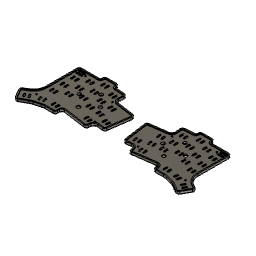
MUSUBI_V2_CASE_SOLID (Autodesk Fusion 360 design; units mm, degrees)
Autodesk Fusion 360 part; units mm, degrees
sketch "WIP_case_bottom" plane through (0, 0, 0) normal (0, 0, 1) x (1, 0, 0)
  arc A0 (118.3392, 82.5249) -> (115.7392, 82.5249) centre (117.0392, 82.5249) ccw
  arc A1 (44.5211, 69.8152) -> (47.0958, 70.177) centre (45.8084, 69.9961) cw
  line L0 (97.2392, 72.1249) -> (97.2392, 67.21)
  line L1 (85.5392, 93.21) -> (85.5392, 98.1249)
  line L2 (134.3532, 17.2954) -> (131.8958, 13.039)
  arc A2 (41.0427, 45.7043) -> (43.6174, 46.0661) centre (42.3301, 45.8852) ccw
  arc A3 (59.8359, 47.9392) -> (62.4296, 48.1205) centre (61.1327, 48.0298) ccw
  line L3 (92.9859, 25.8609) -> (92.9859, 20.9461)
  line L4 (99.7859, 20.9461) -> (99.7859, 25.8609)
  arc A4 (122.5392, 45.5377) -> (125.1392, 45.5377) centre (123.8392, 45.5377) cw
  arc A5 (22.857, 38.5814) -> (25.4317, 38.9432) centre (24.1444, 38.7623) ccw
  arc A6 (88.1392, 56.2105) -> (85.5392, 56.2105) centre (86.8392, 56.2105) cw
  arc A7 (122.5392, 82.5249) -> (125.1392, 82.5249) centre (123.8392, 82.5249) cw
  line L5 (88.1392, 79.6249) -> (88.1392, 74.71)
  line L6 (118.3392, 77.61) -> (118.3392, 82.5249)
  arc A8 (118.3392, 64.0249) -> (115.7392, 64.0249) centre (117.0392, 64.0249) ccw
  line L7 (65.3312, 66.834) -> (64.9884, 71.7369)
  line L8 (104.0392, 48.9605) -> (104.0392, 53.8754)
  arc A9 (125.1392, 59.11) -> (122.5392, 59.11) centre (123.8392, 59.11) cw
  line L9 (106.6392, 53.8754) -> (106.6392, 48.9605)
  line L10 (78.7392, 79.6249) -> (78.7392, 74.71)
  arc A10 (57.2561, 84.8317) -> (59.8498, 85.013) centre (58.5529, 84.9223) ccw
  line L11 (99.8392, 85.71) -> (99.8392, 90.6249)
  arc A11 (95.5859, 25.8609) -> (92.9859, 25.8609) centre (94.2859, 25.8609) ccw
  arc A12 (104.0392, 53.8754) -> (106.6392, 53.8754) centre (105.3392, 53.8754) cw
  arc A13 (140.0364, 8.339) -> (137.7847, 9.639) centre (138.9106, 8.989) cw
  arc A14 (45.5088, 32.6083) -> (42.9341, 32.2464) centre (44.2215, 32.4273) ccw
  line L12 (81.3392, 74.71) -> (81.3392, 79.6249)
  line L13 (52.2427, 33.5546) -> (52.9267, 28.6876)
  arc A15 (102.3859, 20.9461) -> (99.7859, 20.9461) centre (101.0859, 20.9461) cw
  line L14 (61.1415, 66.541) -> (60.7986, 71.4439)
  arc A16 (120.8016, 22.5413) -> (123.313, 21.8684) centre (122.0573, 22.2048) cw
  line L15 (62.4296, 48.1205) -> (62.0867, 53.0234)
  arc A17 (67.9249, 67.0154) -> (65.3312, 66.834) centre (66.6281, 66.9247) cw
  line L16 (78.7392, 98.1249) -> (78.7392, 93.21)
  arc A18 (59.5069, 89.9159) -> (56.9132, 89.7345) centre (58.2101, 89.8252) ccw
  line L17 (118.3392, 59.11) -> (118.3392, 64.0249)
  arc A19 (99.7859, 25.8609) -> (102.3859, 25.8609) centre (101.0859, 25.8609) cw
  arc A20 (115.7392, 40.6228) -> (118.3392, 40.6228) centre (117.0392, 40.6228) ccw
  line L18 (125.1392, 45.5377) -> (125.1392, 40.6228)
  line L19 (104.0392, 67.21) -> (104.0392, 72.1249)
  line L20 (59.8498, 85.013) -> (59.5069, 89.9159)
  arc A21 (140.2422, 13.8954) -> (142.4938, 12.5954) centre (141.368, 13.2454) cw
  line L21 (67.582, 71.9183) -> (67.9249, 67.0154)
  line L22 (43.6174, 46.0661) -> (42.9334, 50.9332)
  line L23 (41.0459, 64.3636) -> (40.3619, 69.2307)
  line L24 (106.6392, 90.6249) -> (106.6392, 85.71)
  line L25 (88.1392, 98.1249) -> (88.1392, 93.21)
  line L26 (99.8392, 48.9605) -> (99.8392, 53.8754)
  arc A22 (64.9884, 71.7369) -> (67.582, 71.9183) centre (66.2852, 71.8276) cw
  line L27 (106.6392, 72.1249) -> (106.6392, 67.21)
  line L28 (125.1392, 82.5249) -> (125.1392, 77.61)
  arc A23 (78.7392, 56.2105) -> (81.3392, 56.2105) centre (80.0392, 56.2105) ccw
  line L29 (95.5859, 20.9461) -> (95.5859, 25.8609)
  line L30 (102.3859, 25.8609) -> (102.3859, 20.9461)
  line L31 (99.8392, 67.21) -> (99.8392, 72.1249)
  line L32 (64.0395, 85.306) -> (63.6967, 90.2089)
  line L33 (46.1928, 27.7412) -> (45.5088, 32.6083)
  arc A24 (63.6967, 90.2089) -> (66.2903, 90.3903) centre (64.9935, 90.2996) cw
  line L34 (85.5392, 56.2105) -> (85.5392, 61.1254)
  arc A25 (66.2765, 53.3164) -> (68.8701, 53.4978) centre (67.5733, 53.4071) cw
  line L35 (115.7392, 45.5377) -> (115.7392, 40.6228)
  line L36 (137.7847, 9.639) -> (140.2422, 13.8954)
  arc A26 (58.5478, 66.3597) -> (61.1415, 66.541) centre (59.8446, 66.4503) ccw
  line L37 (22.173, 43.4484) -> (22.857, 38.5814)
  arc A27 (112.9613, 19.5538) -> (115.4727, 18.8809) centre (114.217, 19.2174) ccw
  arc A28 (52.9267, 28.6876) -> (50.352, 28.3257) centre (51.6393, 28.5067) cw
  arc A29 (88.1392, 74.71) -> (85.5392, 74.71) centre (86.8392, 74.71) cw
  line L38 (97.2392, 90.6249) -> (97.2392, 85.71)
  line L39 (115.7392, 64.0249) -> (115.7392, 59.11)
  arc A30 (62.0867, 53.0234) -> (59.493, 52.842) centre (60.7899, 52.9327) ccw
  arc A31 (104.0392, 90.6249) -> (106.6392, 90.6249) centre (105.3392, 90.6249) cw
  line L40 (42.9341, 32.2464) -> (43.6181, 27.3794)
  arc A32 (47.0926, 51.5177) -> (49.6673, 51.8795) centre (48.3799, 51.6986) cw
  line L41 (85.5392, 74.71) -> (85.5392, 79.6249)
  arc A33 (69.213, 48.5949) -> (66.6193, 48.4135) centre (67.9162, 48.5042) cw
  line L42 (104.0392, 85.71) -> (104.0392, 90.6249)
  line L43 (25.4317, 38.9432) -> (24.7477, 43.8102)
  arc A34 (78.7392, 93.21) -> (81.3392, 93.21) centre (80.0392, 93.21) ccw
  arc A35 (118.3392, 45.5377) -> (115.7392, 45.5377) centre (117.0392, 45.5377) ccw
  arc A36 (49.668, 33.1928) -> (52.2427, 33.5546) centre (50.9553, 33.3737) cw
  arc A37 (88.1392, 93.21) -> (85.5392, 93.21) centre (86.8392, 93.21) cw
  line L44 (59.493, 52.842) -> (59.8359, 47.9392)
  line L45 (122.5392, 77.61) -> (122.5392, 82.5249)
  arc A38 (85.5392, 61.1254) -> (88.1392, 61.1254) centre (86.8392, 61.1254) cw
  line L46 (97.2392, 53.8754) -> (97.2392, 48.9605)
  line L47 (66.2903, 90.3903) -> (66.6332, 85.4874)
  arc A39 (97.2392, 48.9605) -> (99.8392, 48.9605) centre (98.5392, 48.9605) ccw
  arc A40 (47.7798, 65.31) -> (45.2051, 64.9481) centre (46.4924, 65.1291) cw
  line L48 (115.7392, 82.5249) -> (115.7392, 77.61)
  line L49 (66.6193, 48.4135) -> (66.2765, 53.3164)
  arc A41 (106.6392, 67.21) -> (104.0392, 67.21) centre (105.3392, 67.21) cw
  arc A42 (40.3619, 69.2307) -> (37.7872, 68.8688) centre (39.0746, 69.0497) ccw
  line L50 (115.4727, 18.8809) -> (116.7447, 23.6283)
  arc A43 (106.6392, 48.9605) -> (104.0392, 48.9605) centre (105.3392, 48.9605) cw
  arc A44 (125.1392, 77.61) -> (122.5392, 77.61) centre (123.8392, 77.61) cw
  line L51 (122.5392, 59.11) -> (122.5392, 64.0249)
  line L52 (119.5296, 17.7939) -> (120.8016, 22.5413)
  arc A45 (81.3392, 79.6249) -> (78.7392, 79.6249) centre (80.0392, 79.6249) ccw
  arc A46 (85.5392, 98.1249) -> (88.1392, 98.1249) centre (86.8392, 98.1249) cw
  arc A47 (99.8392, 90.6249) -> (97.2392, 90.6249) centre (98.5392, 90.6249) ccw
  arc A48 (115.7392, 77.61) -> (118.3392, 77.61) centre (117.0392, 77.61) ccw
  line L53 (142.4938, 12.5954) -> (140.0364, 8.339)
  line L54 (56.9132, 89.7345) -> (57.2561, 84.8317)
  arc A49 (122.5392, 64.0249) -> (125.1392, 64.0249) centre (123.8392, 64.0249) cw
  arc A50 (115.7392, 59.11) -> (118.3392, 59.11) centre (117.0392, 59.11) ccw
  line L55 (114.2333, 24.3012) -> (112.9613, 19.5538)
  arc A51 (81.3392, 98.1249) -> (78.7392, 98.1249) centre (80.0392, 98.1249) ccw
  line L56 (68.8701, 53.4978) -> (69.213, 48.5949)
  line L57 (81.3392, 56.2105) -> (81.3392, 61.1254)
  arc A52 (32.1656, 39.8896) -> (29.5909, 39.5277) centre (30.8782, 39.7086) cw
  arc A53 (24.7477, 43.8102) -> (22.173, 43.4484) centre (23.4604, 43.6293) ccw
  arc A54 (97.2392, 85.71) -> (99.8392, 85.71) centre (98.5392, 85.71) ccw
  arc A55 (116.7447, 23.6283) -> (114.2333, 24.3012) centre (115.489, 23.9648) ccw
  line L58 (47.7766, 46.6506) -> (47.0926, 51.5177)
  arc A56 (66.6332, 85.4874) -> (64.0395, 85.306) centre (65.3364, 85.3967) cw
  arc A57 (104.0392, 72.1249) -> (106.6392, 72.1249) centre (105.3392, 72.1249) cw
  line L59 (45.2051, 64.9481) -> (44.5211, 69.8152)
  arc A58 (99.8392, 72.1249) -> (97.2392, 72.1249) centre (98.5392, 72.1249) ccw
  arc A59 (38.4712, 64.0018) -> (41.0459, 64.3636) centre (39.7586, 64.1827) ccw
  arc A60 (42.9334, 50.9332) -> (40.3587, 50.5713) centre (41.6461, 50.7522) ccw
  line L60 (125.1392, 64.0249) -> (125.1392, 59.11)
  line L61 (40.3587, 50.5713) -> (41.0427, 45.7043)
  arc A61 (92.9859, 20.9461) -> (95.5859, 20.9461) centre (94.2859, 20.9461) ccw
  line L62 (31.4816, 44.7566) -> (32.1656, 39.8896)
  line L63 (118.3392, 40.6228) -> (118.3392, 45.5377)
  arc A62 (122.041, 17.121) -> (119.5296, 17.7939) centre (120.7853, 17.4574) cw
  arc A63 (97.2392, 67.21) -> (99.8392, 67.21) centre (98.5392, 67.21) ccw
  arc A64 (43.6181, 27.3794) -> (46.1928, 27.7412) centre (44.9055, 27.5603) ccw
  line L64 (47.0958, 70.177) -> (47.7798, 65.31)
  arc A65 (60.7986, 71.4439) -> (58.2049, 71.2625) centre (59.5018, 71.3532) ccw
  line L65 (88.1392, 61.1254) -> (88.1392, 56.2105)
  arc A66 (106.6392, 85.71) -> (104.0392, 85.71) centre (105.3392, 85.71) cw
  line L66 (37.7872, 68.8688) -> (38.4712, 64.0018)
  arc A67 (78.7392, 74.71) -> (81.3392, 74.71) centre (80.0392, 74.71) ccw
  line L67 (58.2049, 71.2625) -> (58.5478, 66.3597)
  line L68 (122.5392, 40.6228) -> (122.5392, 45.5377)
  line L69 (50.352, 28.3257) -> (49.668, 33.1928)
  arc A68 (81.3392, 61.1254) -> (78.7392, 61.1254) centre (80.0392, 61.1254) ccw
  line L70 (78.7392, 61.1254) -> (78.7392, 56.2105)
  arc A69 (50.3513, 47.0125) -> (47.7766, 46.6506) centre (49.0639, 46.8316) cw
  arc A70 (131.8958, 13.039) -> (134.1474, 11.739) centre (133.0216, 12.389) ccw
  line L71 (29.5909, 39.5277) -> (28.9069, 44.3948)
  arc A71 (28.9069, 44.3948) -> (31.4816, 44.7566) centre (30.1942, 44.5757) cw
  arc A72 (125.1392, 40.6228) -> (122.5392, 40.6228) centre (123.8392, 40.6228) cw
  arc A73 (99.8392, 53.8754) -> (97.2392, 53.8754) centre (98.5392, 53.8754) ccw
  line L72 (134.1474, 11.739) -> (136.6049, 15.9954)
  line L73 (81.3392, 93.21) -> (81.3392, 98.1249)
  arc A74 (136.6049, 15.9954) -> (134.3532, 17.2954) centre (135.479, 16.6454) ccw
  line L74 (49.6673, 51.8795) -> (50.3513, 47.0125)
  arc A75 (85.5392, 79.6249) -> (88.1392, 79.6249) centre (86.8392, 79.6249) cw
  line L75 (123.313, 21.8684) -> (122.041, 17.121)
  arc A76 (149.9758, 14.4546) -> (149.2438, 17.1867) centre (148.2438, 15.4546) ccw
  arc A77 (38.4354, 24.3772) -> (29.4001, 31.1861) centre (30.5133, 23.2639) ccw
  line L76 (35.0406, 32.149) -> (36.3397, 29.899)
  circle A78 centre (92.8808, 60.1463) radius 3.2
  line L77 (97.6892, 97.976) -> (128.6892, 97.976)
  line L78 (131.4373, 20.399) -> (132.7363, 22.649)
  line L79 (50.8392, 75.1493) -> (53.4373, 75.1493)
  circle A79 centre (114.7682, 92.976) radius 1.3
  line L80 (36.3397, 34.399) -> (35.0406, 32.149)
  line L81 (128.8392, 24.899) -> (127.5401, 22.649)
  line L82 (53.4373, 79.6493) -> (50.8392, 79.6493)
  line L83 (141.7258, 0.1652) -> (149.9758, 14.4546)
  line L84 (41.2571, 18.6704) -> (80.6009, 24.1996)
  arc A80 (130.6892, 95.976) -> (128.6892, 97.976) centre (128.6892, 95.976) ccw
  line L85 (40.2368, 32.149) -> (38.9378, 34.399)
  arc A81 (93.6892, 101.976) -> (97.6892, 97.976) centre (97.6892, 101.976) ccw
  arc A82 (87.4359, 18.258) -> (80.6009, 24.1996) centre (81.4359, 18.258) ccw
  line L86 (38.9982, 20.3726) -> (38.4354, 24.3772)
  line L87 (36.3397, 29.899) -> (38.9378, 29.899)
  line L88 (127.7922, 89.3705) -> (119.0802, 89.3705)
  arc A83 (119.0802, 96.576) -> (119.0802, 93.976) centre (119.0802, 95.276) ccw
  line L89 (121.0068, 8.8736) -> (109.7331, 11.8943)
  arc A84 (130.6892, 41.7555) -> (142.6892, 20.9709) centre (154.6892, 41.7555) ccw
  arc A85 (127.7922, 93.976) -> (127.7922, 96.576) centre (127.7922, 95.276) ccw
  line L90 (69.4682, 97.9815) -> (52.8591, 96.8201)
  line L91 (49.5401, 77.3993) -> (50.8392, 75.1493)
  line L92 (73.1892, 101.9718) -> (73.1892, 103.476)
  line L93 (138.9938, -0.5669) -> (126.7953, 6.4759)
  line L94 (113.4692, 95.226) -> (112.1701, 92.976)
  line L95 (149.2438, 17.1867) -> (142.6892, 20.9709)
  circle A86 centre (73.1925, 78.5273) radius 3.2
  arc A87 (109.7331, 11.8943) -> (103.5216, 12.712) centre (103.5216, -11.288) ccw
  arc A88 (75.1892, 105.476) -> (73.1892, 103.476) centre (75.1892, 103.476) ccw
  line L96 (127.7922, 96.576) -> (119.0802, 96.576)
  line L97 (132.7363, 22.649) -> (131.4373, 24.899)
  circle A89 centre (74.5198, 40.4393) radius 3.2
  arc A90 (87.4359, 14.712) -> (89.4359, 12.712) centre (89.4359, 14.712) ccw
  line L98 (29.4001, 31.1861) -> (20.4874, 29.9337)
  line L99 (38.9378, 29.899) -> (40.2368, 32.149)
  line L100 (112.1701, 92.976) -> (113.4692, 90.726)
  arc A91 (127.7922, 91.9705) -> (127.7922, 89.3705) centre (127.7922, 90.6705) cw
  circle A92 centre (52.1382, 77.3993) radius 1.3
  line L101 (54.7363, 77.3993) -> (53.4373, 79.6493)
  line L102 (127.5401, 22.649) -> (128.8392, 20.399)
  line L103 (44.761, 77.2722) -> (14.4336, 73.0101)
  line L104 (75.1892, 105.476) -> (91.6892, 105.476)
  arc A93 (93.6892, 103.476) -> (91.6892, 105.476) centre (91.6892, 103.476) ccw
  line L105 (119.0802, 91.9705) -> (127.7922, 91.9705)
  line L106 (38.9378, 34.399) -> (36.3397, 34.399)
  circle A94 centre (130.1382, 22.649) radius 1.3
  line L107 (117.3663, 92.976) -> (116.0673, 95.226)
  line L108 (93.6892, 103.476) -> (93.6892, 101.976)
  line L109 (130.6892, 41.7555) -> (130.6892, 95.976)
  circle A95 centre (54.8122, 58.8197) radius 3.2
  line L110 (116.0673, 95.226) -> (113.4692, 95.226)
  line L111 (53.4373, 75.1493) -> (54.7363, 77.3993)
  arc A96 (69.4682, 97.9815) -> (73.1892, 101.9718) centre (69.1892, 101.9718) ccw
  arc A97 (44.761, 77.2722) -> (51.6282, 85.7524) centre (43.6476, 85.1944) ccw
  arc A98 (52.8591, 96.8201) -> (51.0035, 94.6855) centre (52.9986, 94.825) ccw
  circle A99 centre (73.8502, 59.4845) radius 20.55
  line L112 (116.0673, 90.726) -> (117.3663, 92.976)
  line L113 (50.8392, 79.6493) -> (49.5401, 77.3993)
  line L114 (87.4359, 14.712) -> (87.4359, 18.258)
  line L115 (12.9472, 69.2162) -> (12.7314, 70.7512)
  line L116 (113.4692, 90.726) -> (116.0673, 90.726)
  arc A100 (138.9938, -0.5669) -> (141.7258, 0.1652) centre (139.9938, 1.1652) ccw
  line L117 (119.0802, 93.976) -> (127.7922, 93.976)
  arc A101 (14.4336, 73.0101) -> (12.7314, 70.7512) centre (14.712, 71.0296) ccw
  arc A102 (119.0802, 89.3705) -> (119.0802, 91.9705) centre (119.0802, 90.6705) cw
  arc A103 (38.9982, 20.3726) -> (41.2571, 18.6704) centre (40.9788, 20.6509) ccw
  arc A104 (126.7953, 6.4759) -> (121.0068, 8.8736) centre (114.7953, -14.3087) ccw
  line L118 (131.4373, 24.899) -> (128.8392, 24.899)
  line L119 (51.6282, 85.7524) -> (51.0035, 94.6855)
  circle A105 centre (37.6387, 32.149) radius 1.3
  arc A106 (18.2286, 31.6359) -> (20.4874, 29.9337) centre (20.2091, 31.9142) ccw
  line L120 (103.5216, 12.712) -> (89.4359, 12.712)
  line L121 (128.8392, 20.399) -> (131.4373, 20.399)
  line L122 (95.6892, 103.476) -> (95.6892, 101.976)
  line L123 (12.9472, 69.2162) -> (18.2286, 31.6359)
  line L124 (29.6784, 29.2056) -> (20.7658, 27.9532)
  arc A107 (16.2481, 31.3576) -> (20.7658, 27.9532) centre (20.2091, 31.9142) ccw
  line L125 (10.9666, 68.9379) -> (16.2481, 31.3576)
  line L126 (10.9666, 68.9379) -> (10.7509, 70.4729)
  arc A108 (14.1553, 74.9906) -> (10.7509, 70.4729) centre (14.712, 71.0296) ccw
  line L127 (44.4827, 79.2528) -> (14.1553, 74.9906)
  arc A109 (44.4827, 79.2528) -> (49.633, 85.6129) centre (43.6476, 85.1944) ccw
  line L128 (49.633, 85.6129) -> (49.0084, 94.5459)
  arc A110 (52.7196, 98.8152) -> (49.0084, 94.5459) centre (52.9986, 94.825) ccw
  line L129 (69.3287, 99.9767) -> (52.7196, 98.8152)
  arc A111 (69.3287, 99.9767) -> (71.1892, 101.9718) centre (69.1892, 101.9718) ccw
  line L130 (71.1892, 101.9718) -> (71.1892, 103.476)
  arc A112 (75.1892, 107.476) -> (71.1892, 103.476) centre (75.1892, 103.476) ccw
  line L131 (75.1892, 107.476) -> (91.6892, 107.476)
  arc A113 (95.6892, 103.476) -> (91.6892, 107.476) centre (91.6892, 103.476) ccw
  line L132 (95.6892, 103.476) -> (95.6892, 101.976)
  arc A114 (95.6892, 101.976) -> (97.6892, 99.976) centre (97.6892, 101.976) ccw
  line L133 (97.6892, 99.976) -> (128.6892, 99.976)
  arc A115 (132.6892, 95.976) -> (128.6892, 99.976) centre (128.6892, 95.976) ccw
  line L134 (132.6892, 41.7555) -> (132.6892, 95.976)
  arc A116 (132.6892, 41.7555) -> (143.6892, 22.703) centre (154.6892, 41.7555) ccw
  line L135 (150.2438, 18.9187) -> (143.6892, 22.703)
  arc A117 (151.7079, 13.4546) -> (150.2438, 18.9187) centre (148.2438, 15.4546) ccw
  line L136 (143.4579, -0.8348) -> (151.7079, 13.4546)
  arc A118 (137.9938, -2.2989) -> (143.4579, -0.8348) centre (139.9938, 1.1652) ccw
  line L137 (137.9938, -2.2989) -> (125.7953, 4.7439)
  arc A119 (125.7953, 4.7439) -> (120.4892, 6.9417) centre (114.7953, -14.3087) ccw
  line L138 (120.4892, 6.9417) -> (109.2155, 9.9624)
  arc A120 (109.2155, 9.9624) -> (103.5216, 10.712) centre (103.5216, -11.288) ccw
  line L139 (103.5216, 10.712) -> (89.4359, 10.712)
  arc A121 (85.4359, 14.712) -> (89.4359, 10.712) centre (89.4359, 14.712) ccw
  line L140 (85.4359, 14.712) -> (85.4359, 18.258)
  arc A122 (85.4359, 18.258) -> (80.8792, 22.2191) centre (81.4359, 18.258) ccw
  line L141 (41.5354, 16.6898) -> (80.8792, 22.2191)
  arc A123 (37.0177, 20.0942) -> (41.5354, 16.6898) centre (40.9788, 20.6509) ccw
  line L142 (37.0177, 20.0942) -> (36.4549, 24.0989)
  arc A124 (36.4549, 24.0989) -> (29.6784, 29.2056) centre (30.5133, 23.2639) ccw
  dimension "d28" = 2
  constraint tangent A106 L123
extrude "Extrude1" add sketch "WIP_case_bottom" along normal blind 4.6 contours L122 L124 A107 L125 L126 A108 L127 A109 L128 A110 L129 A111 L130 A112 L131 A113 L132 A114 L133 A115 L134 A116 L135 A117 L136 A118 L137 A119 L138 A120 L139 A121 L140 A122 L141 A123 L142 A124 makes body 1
extrude "Extrude2" add sketch "WIP_case_bottom" along normal blind 3 contours L10 L12 A29 L41 A67 A78 A86 A89 A95 A99 | A76 A77 L77 L83 L84 A80 A81 A82 L86 L89 A84 L90 L92 L93 L95 A87 A88 A90 L98 L103 L104 A93 L108 L109 A96 A97 A98 L114 L115 A100 A101 A103 A104 L119 A106 L120 L123 bodies 1
extrude "Extrude3" add sketch "WIP_case_bottom" along normal blind 1.5 contours A0 L6 L48 A48 | A1 A40 L59 L64 | L0 L31 A58 A63 | L1 L25 A37 A46 | L2 A70 L72 A74 | A2 L22 A60 L61 | A3 L15 A30 L44 | L3 A11 L29 A61 | L4 A15 A19 L30 | A4 L18 L68 A72 | A5 L37 L43 A53 | A6 L34 A38 L65 | A7 L28 L45 A44 | L5 A29 L41 A75 A99 | A29 L41 A99 | L10 L12 A45 A99 | L10 L12 A67 A99 | A8 L17 L39 A50 | L7 A17 L21 A22 | L8 L9 A12 A43 | A9 L51 A49 L60 | A10 A18 L20 L54 | L11 L38 A47 A54 | A13 A21 L36 L53 | A14 L33 L40 A64 | L13 A28 A36 L69 | L14 A26 A65 L67 | A16 L52 A62 L75 | L16 A34 A51 L73 | A20 L35 A35 L63 | L19 L27 A41 A57 | L23 A42 A59 L66 | L24 A31 L42 A66 | L26 L46 A39 A73 | A23 L57 A68 L70 | L32 A24 L47 A56 | A25 A33 L49 L56 | A27 L50 L55 A55 | A32 L58 A69 L74 | A52 L62 L71 A71 bodies 1
extrude "Extrude4" cut sketch "WIP_case_bottom" along normal blind 1 contours A3 L15 A30 L44 | A6 L34 A38 L65 | L10 L12 A29 L41 A67 A78 A86 A89 A95 A99 | A29 L41 A99 | L10 L12 A67 A99 | L7 A17 L21 A22 | L14 A26 A65 L67 | A23 L57 A68 L70 | A25 A33 L49 L56 bodies 1
extrude "Extrude5" add sketch "WIP_case_bottom" along normal blind 1.5 contours L88 A91 L105 A102 | A83 A85 L96 L117 bodies 1
extrude "Extrude6" add sketch "WIP_case_bottom" along normal blind 3 contours L76 L80 L85 L87 L99 L106 | L78 L81 L97 L102 L118 L121 | L79 L82 L91 L101 L111 L113 | A79 | L94 L100 L107 L110 L112 L116 | A92 | A94 | A105 bodies 1
extrude "Extrude7" cut sketch "WIP_case_bottom" along normal blind 3 contours A79 | A92 | A94 | A105 bodies 1
extrude "Extrude8" cut sketch "WIP_case_bottom" along normal blind 1.6 contours L76 L80 L85 L87 L99 L106 | L78 L81 L97 L102 L118 L121 | L79 L82 L91 L101 L111 L113 | L94 L100 L107 L110 L112 L116 bodies 1
chamfer "Chamfer1" distance 0.75 angle 45 36 edges at (49.9798, 97.4492, 0) (49.3207, 90.0794, 0) (48.3105, 81.4184, 0) (29.319, 77.1217, 0) (11.5174, 73.4368, 0) (13.4995, 50.9152, 0) (17.8018, 28.7197, 0) (25.2221, 28.5794, 0) (34.1242, 28.0557, 0) (36.7363, 22.0966, 0) (38.5715, 17.4564, 0) (61.2073, 19.4545, 0) (84.0601, 21.2769, 0) (85.4359, 16.485, 0) (86.6075, 11.8836, 0) (96.4788, 10.712, 0) (106.3931, 10.5238, 0) (114.8524, 8.4521, 0) (123.2143, 6.0167, 0) (131.8946, 1.2225, 0) (141.0291, -2.6985, 0) (147.5829, 6.3099, 0) (152.1075, 16.4899, 0) (146.9665, 20.8108, 0) (135.6367, 30.7556, 0) (132.6892, 68.8658, 0) (131.5176, 98.8044, 0) (113.1892, 99.976, 0) (96.275, 100.5618, 0) (95.6892, 102.726, 0) (94.5176, 106.3044, 0) (83.4392, 107.476, 0) (72.3608, 106.3044, 0) (71.1892, 102.7239, 0) (70.6519, 100.6078, 0) (61.0242, 99.396, 0) on bodies 1
mirror "Mirror1" about plane through (0, 0, 0) normal (1, 0, 0) of bodies 1 makes body 2
extrude "Extrude9" add 40 faces at (-87.2726, 57.8488, 1.5) (-79.6059, 57.8488, 1.5) (-86.4059, 76.3483, 1.5) (-79.6059, 77.9866, 1.5) (-80.4726, 94.8483, 1.5) (-86.4059, 96.4866, 1.5) (-98.1059, 87.3483, 1.5) (-105.7726, 87.3483, 1.5) (-104.9059, 70.4866, 1.5) (-98.1059, 70.4866, 1.5) (-117.4726, 79.2483, 1.5) (-123.4059, 79.2483, 1.5) (-124.2726, 60.7483, 1.5) (-116.6059, 60.7483, 1.5) (-121.9842, 91.1038, 1.5) (-121.9842, 95.7093, 1.5) (-98.1059, 50.5988, 1.5) (-105.7726, 52.2371, 1.5) (-117.4726, 42.2611, 1.5) (-124.2726, 42.2611, 1.5) (-140.105, 10.1912, 1.5) (-134.2846, 15.4433, 1.5) (-121.6279, 18.9277, 1.5) (-115.0596, 20.6877, 1.5) (-101.5192, 22.5843, 1.5) (-94.7192, 22.5843, 1.5) (-65.5401, 88.6955, 1.5) (-58.0064, 86.5264, 1.5) (-65.9672, 70.1631, 1.5) (-59.2981, 68.0544, 1.5) (-67.3696, 50.1083, 1.5) (-61.4507, 49.6944, 1.5) (-51.8404, 30.1893, 1.5) (-44.0204, 30.7447, 1.5) (-49.265, 48.5142, 1.5) (-41.445, 49.0696, 1.5) (-46.6935, 66.8117, 1.5) (-39.9597, 65.8653, 1.5) (-30.8513, 43.0136, 1.5) (-24.3455, 40.4449, 1.5) along direction (0, 0, 1) blind 0.5 on bodies 2 bodies 2
delete_body "RemoveBody1" bodies 2
extrude "Extrude10" add 40 faces at (24.3455, 40.4449, 1.5) (30.8513, 43.0136, 1.5) (44.0204, 30.7447, 1.5) (51.8404, 30.1893, 1.5) (41.445, 49.0696, 1.5) (49.265, 48.5142, 1.5) (39.9597, 65.8653, 1.5) (46.6935, 66.8117, 1.5) (58.0064, 86.5264, 1.5) (65.5401, 88.6955, 1.5) (59.2981, 68.0544, 1.5) (65.9672, 70.1631, 1.5) (61.4507, 49.6944, 1.5) (67.3696, 50.1083, 1.5) (79.6059, 57.8488, 1.5) (87.2726, 57.8488, 1.5) (79.6059, 77.9866, 1.5) (86.4059, 76.3483, 1.5) (80.4726, 94.8483, 1.5) (86.4059, 96.4866, 1.5) (98.1059, 87.3483, 1.5) (105.7726, 87.3483, 1.5) (98.1059, 70.4866, 1.5) (104.9059, 70.4866, 1.5) (98.1059, 50.5988, 1.5) (105.7726, 52.2371, 1.5) (94.7192, 22.5843, 1.5) (101.5192, 22.5843, 1.5) (115.0596, 20.6877, 1.5) (121.6279, 18.9277, 1.5) (134.2846, 15.4433, 1.5) (140.105, 10.1912, 1.5) (117.4726, 42.2611, 1.5) (124.2726, 42.2611, 1.5) (116.6059, 60.7483, 1.5) (124.2726, 60.7483, 1.5) (117.4726, 79.2483, 1.5) (123.4059, 79.2483, 1.5) (121.9842, 91.1038, 1.5) (121.9842, 95.7093, 1.5) along direction (0, 0, 1) blind 0.5 on bodies 1 bodies 1
mirror "Mirror2" about plane through (0, 0, 0) normal (1, 0, 0) of bodies 1 makes body 3
